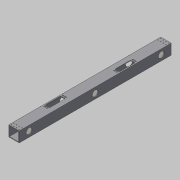
# Autodesk Inventor part: Tube
Saved by Autodesk Inventor 2014 SP1 (Build 180222100, 222)
## iProperties
Created: 2014-01-07
Part Number: Tube
Material: Generic
Document SubType Name: Modeling
Designer: Rauhul Varma
Mass: 399.778 g
Surface Area: 2623.28 cm^2
Volume: 399.778 cm^3
Density: 1 g/cm^3
Appearance: Default
d0: 2.000 in
d1: 2.000 in
d2: 1.750 in
d3: 1.750 in
d4: 0.125 in
d5: 0.125 in
d6: 29.000 in
d7: 0.00 deg
d8: 1.379 in
d9: 0.063 in
d10: 12.598 in
d11: 3.700 in
d12: 1.125 in
d13: 1.125 in
d14: 1.125 in
d15: 1.500 in
d16: 4.199 in
d17: 1.500 in
d18: 4.199 in
d20: 1.938 in
d21: 1.938 in
d22: 1.000 in
d23: 5.799 in
d26: 0.375 in
d27: 0.375 in
d29: 0.286 in
d30: 0.286 in
d33: 0.00 deg
d35: 0.00 deg
d36: 0.063 in
d37: 0.00 deg
d38: 1.469 in
d39: 1.379 in
d40: 1.469 in
d41: 1.379 in
d42: 1.379 in
d43: 1.469 in
d44: 0.591 in
d45: 0.188 in
d46: 0.188 in
d47: 3.000 in
d48: 6.299 in
d54: 0.250 in
d55: 0.250 in
d56: 0.500 in
d57: 0.250 in
d58: 0.250 in
d59: 0.500 in
d60: 2.000 ul
d65: 0.00 deg
d66: 0.125 in
d67: 0.063 in
d68: 0.00 deg
d74: 0.250 in
d75: 0.250 in
d76: 2.000 ul
d78: 0.500 in
d79: 4.000 ul
d81: 0.500 in
d84: 0.125 in
d91: 2.125 in
d92: 0.257 in
d99: 2.125 in
d100: 1.379 in
d101: 0.594 in
r8: 1.125 in
pluglip: 1.938 in
plugdia: 1.500 in
d19: 4.199 in
d24: 5.799 in
d28: 0.286 in
d31: 0.286 in
d49: 6.299 in
d62: 360.00 deg
Author: Rauhul Varma
Autodesk Inventor part; units mm, degrees
note: some values were not read from the file. Chosen so that the rebuilt part matches the saved one: direction of "Rivet Holes"; direction of "Hole2"; direction of "Hole3".
ref_plane "YZ Plane" through (0, 0, 0) normal (1, 0, 0) x (0, 1, 0)
ref_plane "XZ Plane" through (0, 0, 0) normal (0, 1, 0) x (-1, 0, 0)
ref_plane "XY Plane" through (0, 0, 0) normal (0, 0, 1) x (1, 0, 0)
sketch "Sketch1" plane through (0, 0, 0) normal (0, 0, 1) x (1, 0, 0)
  line L0 (0, 0) -> (50.8, 0)
  line L1 (50.8, 0) -> (50.8, 50.8)
  line L2 (50.8, 50.8) -> (0, 50.8)
  line L3 (0, 50.8) -> (0, 0)
  line L4 (3.175, 3.175) -> (47.625, 3.175)
  line L5 (47.625, 3.175) -> (47.625, 47.625)
  line L6 (47.625, 47.625) -> (3.175, 47.625)
  line L7 (3.175, 47.625) -> (3.175, 3.175)
  dimension "d0" = 50.8
  dimension "d1" = 50.8
  dimension "d2" = 44.45
  dimension "d3" = 44.45
  dimension "d4" = 3.175
  dimension "d5" = 3.175
  constraints: 16 end point, 4 parallel, 2 horizontal, 2 perpendicular
  measures "d0" distance of L2.end L1.end
  measures "d1" distance of L1.end L0.end
  measures "d2" distance of L6.end L5.end
  measures "d3" distance of L4.end L5.end
  measures "d4" distance between parallel lines of L2 L6
  measures "d5" distance between parallel lines of L3 L7
extrude "Main Beam" add sketch "Sketch1" along normal mid plane 736.6
sketch "Sketch3" plane through (0, 0, 368.3) normal (-1, 0, 0) x (0, 0, 1)
  line L0 (0, 0) -> (-736.6, 0) projected
  line L1 (0, 50.8) -> (0, 0) projected
  line L2 (-736.6, 50.8) -> (0, 50.8) projected
  line L3 (-736.6, 0) -> (-736.6, 50.8) projected
  line L4 (-368.3, 0) -> (-368.3, 50.8) construction
  line L5 (-736.6, 25.4) -> (0, 25.4) construction
  circle A0 centre (-368.3, 23.8125) radius 17.507 construction
  line L6 (-368.3, 23.8125) -> (-48.3039, 25.4) construction
  circle A1 centre (-48.3039, 25.4) radius 17.507 construction
  circle A2 centre (-48.3039, 25.4) radius 46.99 construction
  line L7 (-1.3139, 79.314) -> (-1.3139, -47.1456) construction
  circle A3 centre (-368.3, 23.8125) radius 14.2875
  circle A4 centre (-48.3039, 25.4) radius 14.2875
  circle A5 centre (-688.2961, 25.4) radius 14.2875
  circle A6 centre (-261.6346, 25.4) radius 19.05
  circle A7 centre (-154.9693, 25.4) radius 19.05
  circle A8 centre (-261.6346, 25.4) radius 24.6063
  circle A9 centre (-154.9693, 25.4) radius 24.6063
  line L8 (-221.002, 50.8) -> (-221.002, 0)
  line L9 (-195.602, 0) -> (-195.602, 50.8)
  circle A10 centre (-130.363, 25.4) radius 4.7625
  circle A11 centre (-286.2409, 25.4) radius 4.7625
  arc A12 (-130.8239, 20.6599) -> (-138.0068, 16.7296) centre (-131.5281, 13.418) ccw
  arc A13 (-138.0068, 34.0704) -> (-130.8239, 30.1401) centre (-131.5281, 37.382) ccw
  arc A14 (-278.5971, 16.7296) -> (-285.78, 20.6599) centre (-285.0759, 13.418) ccw
  arc A15 (-285.78, 30.1401) -> (-278.5971, 34.0704) centre (-285.0759, 37.382) ccw
  point P0 (-368.3, 25.4)
  dimension "d8" = 35.0141
  dimension "d9" = 1.5875
  dimension "d10" = 320
  dimension "d11" = 93.98
  dimension "d12" = 28.575
  dimension "d13" = 28.575
  dimension "d14" = 28.575
  dimension "d15" = 38.1
  dimension "d16" = 106.6654
  dimension "d17" = 38.1
  dimension "d18" = 106.6654
  dimension "d19" = 106.6654
  dimension "d20" = 49.2125
  dimension "d21" = 49.2125
  dimension "d22" = 25.4
  dimension "d23" = 147.298
  dimension "d24" = 147.298
  dimension "d26" = 9.525
  dimension "d27" = 9.525
  dimension "d28" = 7.276
  dimension "d29" = 7.276
  dimension "d30" = 7.276
  dimension "d31" = 7.276
  constraints: 20 point on circle, 16 centre point, 10 end point, 9 tangent, 6 coincident, 5 point on line, 3 midpoint, 2 perpendicular, 1 equal radius, 1 symmetric about line, 1 vertical, 10 other
  measures "d8" diameter of A0
  measures "d10" distance of L6.start L6.end
  measures "d11" diameter of A2
  measures "d12" diameter of A3
  measures "d13" diameter of A4
  measures "d14" diameter of A5
  measures "d15" diameter of A6
  measures "d16" distance from line of L4 A6.centre
  measures "d17" diameter of A7
  measures "d18" distance of A6.centre A7.centre
  measures "d19" distance of L6.end A7.centre
  measures "d20" diameter of A8
  measures "d21" diameter of A9
  measures "d22" distance between parallel lines of L8 L9
  measures "d23" distance between parallel lines of L4 L8
  measures "d24" distance from line of A1.centre L9
  measures "d26" diameter of A10
  measures "d27" diameter of A11
  measures "d28" radius of A12
  measures "d29" radius of A13
  measures "d30" radius of A14
  measures "d31" radius of A15
extrude "Bearing Through Holes" cut sketch "Sketch3" against normal through all contours A3 | A4 | A5
extrude "Access Holes" cut sketch "Sketch3" against normal up to surface (3.175 mm away) contours A6 | A6 A14 A11 A15 | A11 A8 | A8 A11 | A7 | A7 A13 A10 A12 | A10 A9 | A9 A10
extrude "Plug Recesses" cut sketch "Sketch3" against normal blind 1.5875 contours A6 A15 A8 A14 | A6 A14 A11 A15 | A11 A8 | A7 A13 A10 A12 | A7 A12 A9 A13 | A9 A10 picked at (-284.6192, 25.4) picked at (-131.92, 24.4843)
sketch "Sketch4" plane through (0, 50.8, 368.3) normal (0, 1, 0) x (1, 0, 0)
  line L0 (0, 736.6) -> (0, 0) projected
  line L1 (50.8, 0) -> (0, 0) projected
  line L2 (0, 736.6) -> (50.8, 736.6) projected
  line L3 (-10.16, 48.3039) -> (60.96, 48.3039) projected
  line L4 (-10.16, 688.2961) -> (60.96, 688.2961) projected
  line L5 (-10.16, 368.3) -> (60.96, 368.3) projected
  line L6 (25.4, 0) -> (25.4, 736.6) construction
  line L7 (6.7469, 30.7969) -> (44.0531, 30.7969) construction
  line L8 (44.0531, 30.7969) -> (44.0531, 65.811) construction
  line L9 (44.0531, 65.811) -> (6.7469, 65.811) construction
  line L10 (6.7469, 65.811) -> (6.7469, 30.7969) construction
  line L11 (6.7469, 350.793) -> (44.0531, 350.793) construction
  line L12 (44.0531, 350.793) -> (44.0531, 385.807) construction
  line L13 (44.0531, 385.807) -> (6.7469, 385.807) construction
  line L14 (6.7469, 385.807) -> (6.7469, 350.793) construction
  line L15 (6.7469, 705.8031) -> (44.0531, 705.8031) construction
  line L16 (44.0531, 705.8031) -> (44.0531, 670.789) construction
  line L17 (44.0531, 670.789) -> (6.7469, 670.789) construction
  line L18 (6.7469, 670.789) -> (6.7469, 705.8031) construction
  line L19 (8.5734, 30.7969) -> (8.5734, 385.807) construction
  line L20 (23.5734, 385.807) -> (23.5734, 30.7969) construction
  line L21 (16.0734, 65.811) -> (16.0734, 30.7969) construction
  line L22 (0, 246.402) -> (32.1469, 246.402) construction
  line L23 (32.1469, 246.402) -> (32.1469, 170.202) construction
  line L24 (32.1469, 170.202) -> (0, 170.202) construction
  line L25 (0, 170.202) -> (0, 246.402) construction
  line L26 (4.7625, 246.402) -> (4.7625, 170.202)
  line L27 (27.3844, 246.402) -> (27.3844, 170.202)
  line L28 (0, 208.302) -> (32.1469, 208.302) construction
  line L29 (4.7625, 246.402) -> (27.3844, 246.402)
  line L30 (27.3844, 170.202) -> (4.7625, 170.202)
  line L31 (9.7234, 163.852) -> (22.4234, 163.852) construction
  line L32 (9.7234, 160.677) -> (22.4234, 160.677)
  line L33 (22.4234, 167.027) -> (9.7234, 167.027)
  arc A0 (9.7234, 167.027) -> (9.7234, 160.677) centre (9.7234, 163.852) ccw
  arc A1 (22.4234, 160.677) -> (22.4234, 167.027) centre (22.4234, 163.852) ccw
  line L34 (9.7234, 252.752) -> (22.4234, 252.752) construction
  line L35 (9.7234, 249.577) -> (22.4234, 249.577)
  line L36 (22.4234, 255.927) -> (9.7234, 255.927)
  arc A2 (9.7234, 255.927) -> (9.7234, 249.577) centre (9.7234, 252.752) ccw
  arc A3 (22.4234, 249.577) -> (22.4234, 255.927) centre (22.4234, 252.752) ccw
  line L37 (46.0375, 490.198) -> (46.0375, 566.398)
  line L38 (23.4156, 490.198) -> (23.4156, 566.398)
  line L39 (46.0375, 490.198) -> (23.4156, 490.198)
  line L40 (23.4156, 566.398) -> (46.0375, 566.398)
  line L41 (41.0766, 575.923) -> (28.3766, 575.923)
  line L42 (28.3766, 569.573) -> (41.0766, 569.573)
  arc A4 (41.0766, 569.573) -> (41.0766, 575.923) centre (41.0766, 572.748) ccw
  arc A5 (28.3766, 575.923) -> (28.3766, 569.573) centre (28.3766, 572.748) ccw
  line L43 (41.0766, 487.023) -> (28.3766, 487.023)
  line L44 (28.3766, 480.673) -> (41.0766, 480.673)
  arc A6 (41.0766, 480.673) -> (41.0766, 487.023) centre (41.0766, 483.848) ccw
  arc A7 (28.3766, 487.023) -> (28.3766, 480.673) centre (28.3766, 483.848) ccw
  point P0 (0, 368.3)
  point P1 (25.4, 368.3)
  point P2 (16.0734, 163.852)
  point P3 (16.0734, 252.752)
  point P4 (6.35, 6.35)
  point P5 (6.35, 19.05)
  point P6 (19.05, 6.35)
  point P7 (19.05, 19.05)
  point P8 (31.75, 6.35)
  point P9 (31.75, 19.05)
  point P10 (44.45, 6.35)
  point P11 (44.45, 19.05)
  dimension "d38" = 37.3062
  dimension "d39" = 35.0141
  dimension "d40" = 37.3062
  dimension "d41" = 35.0141
  dimension "d42" = 35.0141
  dimension "d43" = 37.3062
  dimension "d44" = 15
  dimension "d45" = 4.7625
  dimension "d46" = 4.7625
  dimension "d47" = 76.2
  dimension "d48" = 159.998
  dimension "d49" = 159.998
  dimension "d54" = 6.35
  dimension "d55" = 6.35
  dimension "d56" = 12.7
  dimension "d57" = 6.35
  dimension "d58" = 6.35
  dimension "d59" = 12.7
  dimension "d62" = 360
  dimension "d74" = 6.35
  dimension "d75" = 6.35
  dimension "d78" = 12.7
  dimension "d81" = 12.7
  constraints: 82 end point, 16 point on circle, 13 parallel, 13 point on line, 9 perpendicular, 8 centre point, 8 tangent, 7 midpoint, 5 horizontal, 1 collinear, 1 vertical, 73 other
  measures "d38" distance between parallel lines of L8 L10
  measures "d39" distance between parallel lines of L9 L7
  measures "d40" distance between parallel lines of L12 L14
  measures "d41" distance between parallel lines of L13 L11
  measures "d42" distance between parallel lines of L17 L15
  measures "d43" distance between parallel lines of L16 L18
  measures "d44" distance between parallel lines of L20 L19
  measures "d45" distance between parallel lines of L25 L26
  measures "d46" distance between parallel lines of L23 L27
  measures "d47" distance of L26.start L26.end
  measures "d48" distance between parallel lines of L3 L28
  measures "d49" distance between parallel lines of L5 L28
  measures "d54" diameter of A1
  measures "d55" distance between parallel lines of L30 L31
  measures "d56" distance of L31.start L31.end
  measures "d57" diameter of A3
  measures "d58" distance between parallel lines of L29 L34
  measures "d59" distance of L34.start L34.end
  measures "d74" distance from line of L1 point (6.35, 6.35)
  measures "d75" distance from line of L0 point (6.35, 6.35)
  measures "d78" distance of point (6.35, 6.35) point (6.35, 19.05)
  measures "d81" distance of point (6.35, 6.35) point (19.05, 6.35)
extrude "Extrusion5" cut sketch "Sketch4" against normal up to surface (3.175 mm away) contours L29 L27 L30 L26 | L39 L38 L40 L37
fillet "Fillet1" radius 3.175 8 edges at (4.7625, 49.2125, 121.898) (27.3844, 49.2125, 121.898) (27.3844, 49.2125, 198.098) (4.7625, 49.2125, 198.098) (23.4156, 49.2125, -198.098) (46.0375, 49.2125, -198.098) (46.0375, 49.2125, -121.898) (23.4156, 49.2125, -121.898)
extrude "Extrusion6" cut sketch "Sketch4" against normal blind 1.5875 contours A0 L33 A1 L32 | A2 L36 A3 L35 | A4 L42 A5 L41 | A6 L44 A7 L43
hole "Rivet Holes" at (6.35, 50.8, 361.95) at (6.35, 50.8, 349.25) at (19.05, 50.8, 361.95) at (19.05, 50.8, 349.25) at (31.75, 50.8, 361.95) at (31.75, 50.8, 349.25) at (44.45, 50.8, 361.95) at (44.45, 50.8, 349.25) direction (0, -1, 0) diameter 3.175 end up to surface
mirror "Mirror1" about plane through (0, 0, 0) normal (0, 0, 1) of "Access Holes", "Plug Recesses", "Rivet Holes"
sketch "Sketch5" plane through (50.8, 0, 368.3) normal (1, 0, 0) x (0, 0, -1)
  circle A0 centre (368.3, 23.8125) radius 14.2875 projected
  circle A1 centre (368.3, 23.8125) radius 26.9875 construction
  line L0 (341.3125, 23.8125) -> (395.2875, 23.8125) construction
  point P0 (368.3, 0)
  dimension "d91" = 53.975
  constraints: 3 coincident, 2 end point, 2 point on circle, 1 centre point, 1 horizontal, 1 midpoint
  measures "d91" diameter of A1
hole "Hole2" at (50.8, 23.8125, 26.9875) at (50.8, 23.8125, -26.9875) direction (-1, 0, 0) diameter 6.5278 end up to surface clearance for "Flat Head Machine Screw (82)" size "1/4" standard "Ansi Unified Screw Threads"
sketch "Sketch6" plane through (0, 0, 368.3) normal (-1, 0, 0) x (0, 0, 1)
  circle A0 centre (-368.3, 23.8125) radius 14.2875 projected
  circle A1 centre (-368.3, 23.8125) radius 26.9875 construction
  circle A2 centre (-368.3, 23.8125) radius 17.507 construction
  line L0 (-395.2875, 23.8125) -> (-341.3125, 23.8125) construction
  point P0 (-368.3, 0)
  dimension "d99" = 53.975
  dimension "d100" = 35.0141
  dimension "d108" = 35.0141
  dimension "d109" = 2.54
  constraints: 4 coincident, 2 centre point, 2 end point, 2 point on circle, 1 horizontal, 1 midpoint
  measures "d99" diameter of A1
  measures "d100" diameter of A2
hole "Hole3" at (0, 23.8125, -26.9875) at (0, 23.8125, 26.9875) direction (1, 0, 0) diameter 15.0812 end up to surface
equation "\"d12\" = r8"
equation "\"d13\" = r8"
equation "\"d14\" = r8"
equation "\"d15\" = plugdia"
equation "\"d16\" = d19"
equation "\"d17\" = plugdia"
equation "\"d18\" = d16"
equation "\"d20\" = pluglip"
equation "\"d21\" = pluglip"
equation "\"d23\" = d24"
equation "\"d29\" = d28"
equation "\"d30\" = d31"
equation "\"d40\" = d38"
equation "\"d41\" = d39"
equation "\"d42\" = d41"
equation "\"d43\" = d40"
equation "\"d46\" = d45"
equation "\"d48\" = d49"
equation "\"d55\" = d54"
equation "\"d58\" = d57"
equation "\"r8\" = 28.575"
equation "\"pluglip\" = 49.2125"
equation "\"plugdia\" = 38.1"
body "Solid1"
